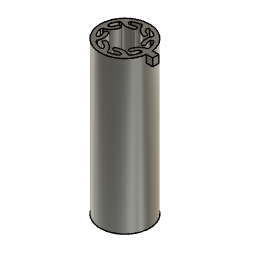
Linear_Bearing_V1.1 v1 (Autodesk Fusion 360 design; units mm, degrees)
Autodesk Fusion 360 part; units mm, degrees
sketch "Sketch1" plane through (0, 0, 0) normal (0, 0, 1) x (1, 0, 0)
  circle A0 centre (0, 0) radius 1.625
  spline S0 degree 5 poles (1.3709, -0.1056) (1.3505, -0.1114) (1.3112, -0.1235) (1.2571, -0.1431) (1.195, -0.1719) (1.1338, -0.2127) (1.088, -0.2577) (1.056, -0.3063) (1.0348, -0.3573) (1.0195, -0.4088) (1.0044, -0.4583) (0.984, -0.5029) (0.9544, -0.5399) (0.9148, -0.5662) (0.8686, -0.5794) (0.8219, -0.5775) (0.7819, -0.5594) (0.755, -0.5253) (0.7447, -0.4768) (0.751, -0.4174) (0.7717, -0.351) (0.8032, -0.2822) (0.8417, -0.2149) (0.8842, -0.1519) (0.9289, -0.0947) (0.9753, -0.0437) (1.0232, 0.0013) (1.0731, 0.0411) (1.1254, 0.0764) (1.1804, 0.1076) (1.2383, 0.135) (1.2869, 0.154) (1.3246, 0.1667) (1.3504, 0.1744) (1.3634, 0.1781) knots 0 0 0 0 0 0 0.033333 0.066667 0.1 0.133333 0.166667 0.2 0.233333 0.266667 0.3 0.333333 0.366667 0.4 0.433333 0.466667 0.5 0.533333 0.566667 0.6 0.633333 0.666667 0.7 0.733333 0.766667 0.8 0.833333 0.866667 0.9 0.933333 0.966667 1 1 1 1 1 1
  spline S1 degree 5 poles (1.0441, 0.8947) (1.0337, 0.8761) (1.0145, 0.8398) (0.9901, 0.7878) (0.9666, 0.7234) (0.9521, 0.6513) (0.9516, 0.5871) (0.9633, 0.5301) (0.9844, 0.479) (1.01, 0.4319) (1.0343, 0.3862) (1.0514, 0.3401) (1.0566, 0.2931) (1.0472, 0.2465) (1.0239, 0.2045) (0.9895, 0.1728) (0.9485, 0.1573) (0.9053, 0.1624) (0.8637, 0.1894) (0.8261, 0.2359) (0.7939, 0.2974) (0.7675, 0.3684) (0.7471, 0.4432) (0.7326, 0.5178) (0.7238, 0.5899) (0.7206, 0.6587) (0.7226, 0.7245) (0.7297, 0.7879) (0.7418, 0.8498) (0.7586, 0.9108) (0.7802, 0.971) (0.8011, 1.0188) (0.8188, 1.0545) (0.8315, 1.0782) (0.8381, 1.09) knots 0 0 0 0 0 0 0.033333 0.066667 0.1 0.133333 0.166667 0.2 0.233333 0.266667 0.3 0.333333 0.366667 0.4 0.433333 0.466667 0.5 0.533333 0.566667 0.6 0.633333 0.666667 0.7 0.733333 0.766667 0.8 0.833333 0.866667 0.9 0.933333 0.966667 1 1 1 1 1 1
  spline S2 degree 5 poles (0.1056, 1.3709) (0.1114, 1.3505) (0.1235, 1.3112) (0.1431, 1.2571) (0.1719, 1.195) (0.2127, 1.1338) (0.2577, 1.088) (0.3063, 1.056) (0.3573, 1.0348) (0.4088, 1.0195) (0.4583, 1.0044) (0.5029, 0.984) (0.5399, 0.9544) (0.5662, 0.9148) (0.5794, 0.8686) (0.5775, 0.8219) (0.5594, 0.7819) (0.5253, 0.755) (0.4768, 0.7447) (0.4174, 0.751) (0.351, 0.7717) (0.2822, 0.8032) (0.2149, 0.8417) (0.1519, 0.8842) (0.0947, 0.9289) (0.0437, 0.9753) (-0.0013, 1.0232) (-0.0411, 1.0731) (-0.0764, 1.1254) (-0.1076, 1.1804) (-0.135, 1.2383) (-0.154, 1.2869) (-0.1667, 1.3246) (-0.1744, 1.3504) (-0.1781, 1.3634) knots 0 0 0 0 0 0 0.033333 0.066667 0.1 0.133333 0.166667 0.2 0.233333 0.266667 0.3 0.333333 0.366667 0.4 0.433333 0.466667 0.5 0.533333 0.566667 0.6 0.633333 0.666667 0.7 0.733333 0.766667 0.8 0.833333 0.866667 0.9 0.933333 0.966667 1 1 1 1 1 1
  spline S3 degree 5 poles (-0.8947, 1.0441) (-0.8761, 1.0337) (-0.8398, 1.0145) (-0.7878, 0.9901) (-0.7234, 0.9666) (-0.6513, 0.9521) (-0.5871, 0.9516) (-0.5301, 0.9633) (-0.479, 0.9844) (-0.4319, 1.01) (-0.3862, 1.0343) (-0.3401, 1.0514) (-0.2931, 1.0566) (-0.2465, 1.0472) (-0.2045, 1.0239) (-0.1728, 0.9895) (-0.1573, 0.9485) (-0.1624, 0.9053) (-0.1894, 0.8637) (-0.2359, 0.8261) (-0.2974, 0.7939) (-0.3684, 0.7675) (-0.4432, 0.7471) (-0.5178, 0.7326) (-0.5899, 0.7238) (-0.6587, 0.7206) (-0.7245, 0.7226) (-0.7879, 0.7297) (-0.8498, 0.7418) (-0.9108, 0.7586) (-0.971, 0.7802) (-1.0188, 0.8011) (-1.0545, 0.8188) (-1.0782, 0.8315) (-1.09, 0.8381) knots 0 0 0 0 0 0 0.033333 0.066667 0.1 0.133333 0.166667 0.2 0.233333 0.266667 0.3 0.333333 0.366667 0.4 0.433333 0.466667 0.5 0.533333 0.566667 0.6 0.633333 0.666667 0.7 0.733333 0.766667 0.8 0.833333 0.866667 0.9 0.933333 0.966667 1 1 1 1 1 1
  spline S4 degree 5 poles (-1.3709, 0.1056) (-1.3505, 0.1114) (-1.3112, 0.1235) (-1.2571, 0.1431) (-1.195, 0.1719) (-1.1338, 0.2127) (-1.088, 0.2577) (-1.056, 0.3063) (-1.0348, 0.3573) (-1.0195, 0.4088) (-1.0044, 0.4583) (-0.984, 0.5029) (-0.9544, 0.5399) (-0.9148, 0.5662) (-0.8686, 0.5794) (-0.8219, 0.5775) (-0.7819, 0.5594) (-0.755, 0.5253) (-0.7447, 0.4768) (-0.751, 0.4174) (-0.7717, 0.351) (-0.8032, 0.2822) (-0.8417, 0.2149) (-0.8842, 0.1519) (-0.9289, 0.0947) (-0.9753, 0.0437) (-1.0232, -0.0013) (-1.0731, -0.0411) (-1.1254, -0.0764) (-1.1804, -0.1076) (-1.2383, -0.135) (-1.2869, -0.154) (-1.3246, -0.1667) (-1.3504, -0.1744) (-1.3634, -0.1781) knots 0 0 0 0 0 0 0.033333 0.066667 0.1 0.133333 0.166667 0.2 0.233333 0.266667 0.3 0.333333 0.366667 0.4 0.433333 0.466667 0.5 0.533333 0.566667 0.6 0.633333 0.666667 0.7 0.733333 0.766667 0.8 0.833333 0.866667 0.9 0.933333 0.966667 1 1 1 1 1 1
  spline S5 degree 5 poles (-1.0441, -0.8947) (-1.0337, -0.8761) (-1.0145, -0.8398) (-0.9901, -0.7878) (-0.9666, -0.7234) (-0.9521, -0.6513) (-0.9516, -0.5871) (-0.9633, -0.5301) (-0.9844, -0.479) (-1.01, -0.4319) (-1.0343, -0.3862) (-1.0514, -0.3401) (-1.0566, -0.2931) (-1.0472, -0.2465) (-1.0239, -0.2045) (-0.9895, -0.1728) (-0.9485, -0.1573) (-0.9053, -0.1624) (-0.8637, -0.1894) (-0.8261, -0.2359) (-0.7939, -0.2974) (-0.7675, -0.3684) (-0.7471, -0.4432) (-0.7326, -0.5178) (-0.7238, -0.5899) (-0.7206, -0.6587) (-0.7226, -0.7245) (-0.7297, -0.7879) (-0.7418, -0.8498) (-0.7586, -0.9108) (-0.7802, -0.971) (-0.8011, -1.0188) (-0.8188, -1.0545) (-0.8315, -1.0782) (-0.8381, -1.09) knots 0 0 0 0 0 0 0.033333 0.066667 0.1 0.133333 0.166667 0.2 0.233333 0.266667 0.3 0.333333 0.366667 0.4 0.433333 0.466667 0.5 0.533333 0.566667 0.6 0.633333 0.666667 0.7 0.733333 0.766667 0.8 0.833333 0.866667 0.9 0.933333 0.966667 1 1 1 1 1 1
  spline S6 degree 5 poles (-0.1056, -1.3709) (-0.1114, -1.3505) (-0.1235, -1.3112) (-0.1431, -1.2571) (-0.1719, -1.195) (-0.2127, -1.1338) (-0.2577, -1.088) (-0.3063, -1.056) (-0.3573, -1.0348) (-0.4088, -1.0195) (-0.4583, -1.0044) (-0.5029, -0.984) (-0.5399, -0.9544) (-0.5662, -0.9148) (-0.5794, -0.8686) (-0.5775, -0.8219) (-0.5594, -0.7819) (-0.5253, -0.755) (-0.4768, -0.7447) (-0.4174, -0.751) (-0.351, -0.7717) (-0.2822, -0.8032) (-0.2149, -0.8417) (-0.1519, -0.8842) (-0.0947, -0.9289) (-0.0437, -0.9753) (0.0013, -1.0232) (0.0411, -1.0731) (0.0764, -1.1254) (0.1076, -1.1804) (0.135, -1.2383) (0.154, -1.2869) (0.1667, -1.3246) (0.1744, -1.3504) (0.1781, -1.3634) knots 0 0 0 0 0 0 0.033333 0.066667 0.1 0.133333 0.166667 0.2 0.233333 0.266667 0.3 0.333333 0.366667 0.4 0.433333 0.466667 0.5 0.533333 0.566667 0.6 0.633333 0.666667 0.7 0.733333 0.766667 0.8 0.833333 0.866667 0.9 0.933333 0.966667 1 1 1 1 1 1
  spline S7 degree 5 poles (0.8947, -1.0441) (0.8761, -1.0337) (0.8398, -1.0145) (0.7878, -0.9901) (0.7234, -0.9666) (0.6513, -0.9521) (0.5871, -0.9516) (0.5301, -0.9633) (0.479, -0.9844) (0.4319, -1.01) (0.3862, -1.0343) (0.3401, -1.0514) (0.2931, -1.0566) (0.2465, -1.0472) (0.2045, -1.0239) (0.1728, -0.9895) (0.1573, -0.9485) (0.1624, -0.9053) (0.1894, -0.8637) (0.2359, -0.8261) (0.2974, -0.7939) (0.3684, -0.7675) (0.4432, -0.7471) (0.5178, -0.7326) (0.5899, -0.7238) (0.6587, -0.7206) (0.7245, -0.7226) (0.7879, -0.7297) (0.8498, -0.7418) (0.9108, -0.7586) (0.971, -0.7802) (1.0188, -0.8011) (1.0545, -0.8188) (1.0782, -0.8315) (1.09, -0.8381) knots 0 0 0 0 0 0 0.033333 0.066667 0.1 0.133333 0.166667 0.2 0.233333 0.266667 0.3 0.333333 0.366667 0.4 0.433333 0.466667 0.5 0.533333 0.566667 0.6 0.633333 0.666667 0.7 0.733333 0.766667 0.8 0.833333 0.866667 0.9 0.933333 0.966667 1 1 1 1 1 1
  arc A1 (1.3634, 0.1781) -> (1.0441, 0.8947) centre (0, 0) ccw
  arc A2 (0.8381, 1.09) -> (0.1056, 1.3709) centre (0, 0) ccw
  arc A3 (-0.1781, 1.3634) -> (-0.8947, 1.0441) centre (0, 0) ccw
  arc A4 (-1.09, 0.8381) -> (-1.3709, 0.1056) centre (0, 0) ccw
  arc A5 (-1.3634, -0.1781) -> (-1.0441, -0.8947) centre (0, 0) ccw
  arc A6 (-0.8381, -1.09) -> (-0.1056, -1.3709) centre (0, 0) ccw
  arc A7 (0.1781, -1.3634) -> (0.8947, -1.0441) centre (0, 0) ccw
  arc A8 (1.09, -0.8381) -> (1.3709, -0.1056) centre (0, 0) ccw
  point P0 (1.0505, -0.323)
  point P1 (0.9486, -0.5402)
  point P2 (0.7669, -0.5357)
  point P3 (0.8289, -0.2388)
  point P4 (1.0683, 0.0359)
  point P5 (0.9713, 0.5144)
  point P6 (1.0527, 0.2888)
  point P7 (0.9211, 0.1635)
  point P8 (0.755, 0.4173)
  point P9 (0.73, 0.7808)
  point P10 (0.323, 1.0505)
  point P11 (0.5402, 0.9486)
  point P12 (0.5357, 0.7669)
  point P13 (0.2388, 0.8289)
  point P14 (-0.0359, 1.0683)
  point P15 (-0.5144, 0.9713)
  point P16 (-0.2888, 1.0527)
  point P17 (-0.1635, 0.9211)
  point P18 (-0.4173, 0.755)
  point P19 (-0.7808, 0.73)
  point P20 (-1.0505, 0.323)
  point P21 (-0.9486, 0.5402)
  point P22 (-0.7669, 0.5357)
  point P23 (-0.8289, 0.2388)
  point P24 (-1.0683, -0.0359)
  point P25 (-0.9713, -0.5144)
  point P26 (-1.0527, -0.2888)
  point P27 (-0.9211, -0.1635)
  point P28 (-0.755, -0.4173)
  point P29 (-0.73, -0.7808)
  point P30 (-0.323, -1.0505)
  point P31 (-0.5402, -0.9486)
  point P32 (-0.5357, -0.7669)
  point P33 (-0.2388, -0.8289)
  point P34 (0.0359, -1.0683)
  point P35 (0.5144, -0.9713)
  point P36 (0.2888, -1.0527)
  point P37 (0.1635, -0.9211)
  point P38 (0.4173, -0.755)
  point P39 (0.7808, -0.73)
  dimension "d1" = 3.25
  dimension "d2" = 2.75
  dimension "d4" = 360
  constraint coincident A0.centre A1.centre
  constraint concentric A1 A2
  constraint concentric A2 A3
  constraint concentric A3 A4
  constraint concentric A4 A5
  constraint concentric A5 A6
  constraint concentric A6 A7
  constraint concentric A7 A8
  measures "d1" diameter of A0
  measures "d2" diameter of A1
extrude "Extrude1" add sketch "Sketch1" along normal blind 10
fillet "Fillet1" radius 0.1 16 edges at (-1.09, 0.8381, 5) (-0.8947, 1.0441, 5) (-1.3634, -0.1781, 5) (-1.3709, 0.1056, 5) (-0.1781, 1.3634, 5) (0.8381, 1.09, 5) (1.3709, -0.1056, 5) (0.1056, 1.3709, 5) (1.0441, 0.8947, 5) (1.3634, 0.1781, 5) (1.09, -0.8381, 5) (0.8947, -1.0441, 5) (0.1781, -1.3634, 5) (-1.0441, -0.8947, 5) (-0.8381, -1.09, 5) (-0.1056, -1.3709, 5)
sketch "Sketch2" plane through (0, 0, 10) normal (0, 0, 1) x (-1, 0, 0)
  arc A0 (-1.1419, 0.7659) -> (-1.346, 0.2807) centre (0, 0) ccw
  spline S0 degree 3 poles (-1.0172, 0.8011) (-1.029, 0.8065) (-1.0418, 0.8096) (-1.0678, 0.8107) (-1.0808, 0.8087) (-1.1029, 0.8006) (-1.1122, 0.7955) (-1.1288, 0.7825) (-1.136, 0.7747) (-1.1419, 0.7659) knots 0 0 0 0 0.003906 0.003906 0.007813 0.007813 0.010976 0.010976 0.01414 0.01414 0.01414 0.01414
  spline S1 degree 5 poles (-1.0172, 0.8011) (-1.0079, 0.7969) (-0.9867, 0.7875) (-0.9535, 0.7739) (-0.908, 0.7579) (-0.8498, 0.7418) (-0.7879, 0.7297) (-0.7245, 0.7226) (-0.6587, 0.7206) (-0.5899, 0.7238) (-0.5178, 0.7326) (-0.4432, 0.7471) (-0.3684, 0.7675) (-0.2974, 0.7939) (-0.2359, 0.8261) (-0.1894, 0.8637) (-0.1624, 0.9053) (-0.1573, 0.9485) (-0.1728, 0.9895) (-0.2045, 1.0239) (-0.2465, 1.0472) (-0.2931, 1.0566) (-0.3401, 1.0514) (-0.3862, 1.0343) (-0.4319, 1.01) (-0.479, 0.9844) (-0.5301, 0.9633) (-0.5871, 0.9516) (-0.6386, 0.952) (-0.6809, 0.9586) (-0.7108, 0.966) (-0.7262, 0.9705) (-0.7264, 0.9706) knots -0.959103 -0.959103 -0.959103 -0.959103 -0.959103 -0.959103 -0.933333 -0.9 -0.866667 -0.833333 -0.8 -0.766667 -0.733333 -0.7 -0.666667 -0.633333 -0.6 -0.566667 -0.533333 -0.5 -0.466667 -0.433333 -0.4 -0.366667 -0.333333 -0.3 -0.266667 -0.233333 -0.2 -0.166667 -0.133333 -0.1 -0.066667 -0.066274 -0.066274 -0.066274 -0.066274 -0.066274 -0.066274
  spline S2 degree 3 poles (-0.7533, 1.1503) (-0.7642, 1.1431) (-0.7736, 1.1339) (-0.7884, 1.1125) (-0.7936, 1.1004) (-0.799, 1.0749) (-0.7993, 1.0618) (-0.7947, 1.0362) (-0.7899, 1.0239) (-0.7764, 1.0027) (-0.7682, 0.9938) (-0.7489, 0.9794) (-0.738, 0.9739) (-0.7264, 0.9706) knots 0 0 0 0 0.003906 0.003906 0.007813 0.007813 0.011719 0.011719 0.015626 0.015626 0.019244 0.019244 0.022863 0.022863 0.022863 0.022863
  arc A1 (-0.2659, 1.3491) -> (-0.7533, 1.1503) centre (0, 0) ccw
  spline S3 degree 3 poles (-0.1528, 1.2857) (-0.1573, 1.2979) (-0.1642, 1.3091) (-0.1818, 1.3283) (-0.1924, 1.336) (-0.2138, 1.346) (-0.224, 1.3489) (-0.2449, 1.3515) (-0.2555, 1.3511) (-0.2659, 1.3491) knots 0 0 0 0 0.003906 0.003906 0.007813 0.007813 0.010976 0.010976 0.01414 0.01414 0.01414 0.01414
  spline S4 degree 5 poles (-0.1528, 1.2857) (-0.1492, 1.2762) (-0.1409, 1.2546) (-0.127, 1.2215) (-0.1061, 1.1779) (-0.0764, 1.1254) (-0.0411, 1.0731) (-0.0013, 1.0232) (0.0437, 0.9753) (0.0947, 0.9289) (0.1519, 0.8842) (0.2149, 0.8417) (0.2822, 0.8032) (0.351, 0.7717) (0.4174, 0.751) (0.4768, 0.7447) (0.5253, 0.755) (0.5594, 0.7819) (0.5775, 0.8219) (0.5794, 0.8686) (0.5662, 0.9148) (0.5399, 0.9544) (0.5029, 0.984) (0.4583, 1.0044) (0.4088, 1.0195) (0.3573, 1.0348) (0.3063, 1.056) (0.2577, 1.088) (0.2216, 1.1247) (0.1964, 1.1593) (0.1805, 1.1857) (0.1727, 1.1998) (0.1726, 1.1999) knots -0.959103 -0.959103 -0.959103 -0.959103 -0.959103 -0.959103 -0.933333 -0.9 -0.866667 -0.833333 -0.8 -0.766667 -0.733333 -0.7 -0.666667 -0.633333 -0.6 -0.566667 -0.533333 -0.5 -0.466667 -0.433333 -0.4 -0.366667 -0.333333 -0.3 -0.266667 -0.233333 -0.2 -0.166667 -0.133333 -0.1 -0.066667 -0.066274 -0.066274 -0.066274 -0.066274 -0.066274 -0.066274
  spline S5 degree 3 poles (0.2807, 1.346) (0.2679, 1.3487) (0.2548, 1.3488) (0.2292, 1.3441) (0.217, 1.3392) (0.1951, 1.3251) (0.1856, 1.316) (0.1707, 1.2946) (0.1655, 1.2826) (0.16, 1.2581) (0.1596, 1.2459) (0.163, 1.222) (0.1668, 1.2105) (0.1726, 1.1999) knots 0 0 0 0 0.003906 0.003906 0.007813 0.007813 0.011719 0.011719 0.015626 0.015626 0.019244 0.019244 0.022863 0.022863 0.022863 0.022863
  arc A2 (0.7659, 1.1419) -> (0.2807, 1.346) centre (0, 0) ccw
  spline S6 degree 3 poles (0.8011, 1.0172) (0.8065, 1.029) (0.8096, 1.0418) (0.8107, 1.0678) (0.8087, 1.0808) (0.8006, 1.1029) (0.7955, 1.1122) (0.7825, 1.1288) (0.7747, 1.136) (0.7659, 1.1419) knots 0 0 0 0 0.003906 0.003906 0.007813 0.007813 0.010976 0.010976 0.01414 0.01414 0.01414 0.01414
  spline S7 degree 5 poles (0.8011, 1.0172) (0.7969, 1.0079) (0.7875, 0.9867) (0.7739, 0.9535) (0.7579, 0.908) (0.7418, 0.8498) (0.7297, 0.7879) (0.7226, 0.7245) (0.7206, 0.6587) (0.7238, 0.5899) (0.7326, 0.5178) (0.7471, 0.4432) (0.7675, 0.3684) (0.7939, 0.2974) (0.8261, 0.2359) (0.8637, 0.1894) (0.9053, 0.1624) (0.9485, 0.1573) (0.9895, 0.1728) (1.0239, 0.2045) (1.0472, 0.2465) (1.0566, 0.2931) (1.0514, 0.3401) (1.0343, 0.3862) (1.01, 0.4319) (0.9844, 0.479) (0.9633, 0.5301) (0.9516, 0.5871) (0.952, 0.6386) (0.9586, 0.6809) (0.966, 0.7108) (0.9705, 0.7262) (0.9706, 0.7264) knots -0.959103 -0.959103 -0.959103 -0.959103 -0.959103 -0.959103 -0.933333 -0.9 -0.866667 -0.833333 -0.8 -0.766667 -0.733333 -0.7 -0.666667 -0.633333 -0.6 -0.566667 -0.533333 -0.5 -0.466667 -0.433333 -0.4 -0.366667 -0.333333 -0.3 -0.266667 -0.233333 -0.2 -0.166667 -0.133333 -0.1 -0.066667 -0.066274 -0.066274 -0.066274 -0.066274 -0.066274 -0.066274
  spline S8 degree 3 poles (1.1503, 0.7533) (1.1431, 0.7642) (1.1339, 0.7736) (1.1125, 0.7884) (1.1004, 0.7936) (1.0749, 0.799) (1.0618, 0.7993) (1.0362, 0.7947) (1.0239, 0.7899) (1.0027, 0.7764) (0.9938, 0.7682) (0.9794, 0.7489) (0.9739, 0.738) (0.9706, 0.7264) knots 0 0 0 0 0.003906 0.003906 0.007813 0.007813 0.011719 0.011719 0.015626 0.015626 0.019244 0.019244 0.022863 0.022863 0.022863 0.022863
  arc A3 (1.3491, 0.2659) -> (1.1503, 0.7533) centre (0, 0) ccw
  spline S9 degree 3 poles (1.2857, 0.1528) (1.2979, 0.1573) (1.3091, 0.1642) (1.3283, 0.1818) (1.336, 0.1924) (1.346, 0.2138) (1.3489, 0.224) (1.3515, 0.2449) (1.3511, 0.2555) (1.3491, 0.2659) knots 0 0 0 0 0.003906 0.003906 0.007813 0.007813 0.010976 0.010976 0.01414 0.01414 0.01414 0.01414
  spline S10 degree 5 poles (1.2857, 0.1528) (1.2762, 0.1492) (1.2546, 0.1409) (1.2215, 0.127) (1.1779, 0.1061) (1.1254, 0.0764) (1.0731, 0.0411) (1.0232, 0.0013) (0.9753, -0.0437) (0.9289, -0.0947) (0.8842, -0.1519) (0.8417, -0.2149) (0.8032, -0.2822) (0.7717, -0.351) (0.751, -0.4174) (0.7447, -0.4768) (0.755, -0.5253) (0.7819, -0.5594) (0.8219, -0.5775) (0.8686, -0.5794) (0.9148, -0.5662) (0.9544, -0.5399) (0.984, -0.5029) (1.0044, -0.4583) (1.0195, -0.4088) (1.0348, -0.3573) (1.056, -0.3063) (1.088, -0.2577) (1.1247, -0.2216) (1.1593, -0.1964) (1.1857, -0.1805) (1.1998, -0.1727) (1.1999, -0.1726) knots -0.959103 -0.959103 -0.959103 -0.959103 -0.959103 -0.959103 -0.933333 -0.9 -0.866667 -0.833333 -0.8 -0.766667 -0.733333 -0.7 -0.666667 -0.633333 -0.6 -0.566667 -0.533333 -0.5 -0.466667 -0.433333 -0.4 -0.366667 -0.333333 -0.3 -0.266667 -0.233333 -0.2 -0.166667 -0.133333 -0.1 -0.066667 -0.066274 -0.066274 -0.066274 -0.066274 -0.066274 -0.066274
  spline S11 degree 3 poles (1.346, -0.2807) (1.3487, -0.2679) (1.3488, -0.2548) (1.3441, -0.2292) (1.3392, -0.217) (1.3251, -0.1951) (1.316, -0.1856) (1.2946, -0.1707) (1.2826, -0.1655) (1.2581, -0.16) (1.2459, -0.1596) (1.222, -0.163) (1.2105, -0.1668) (1.1999, -0.1726) knots 0 0 0 0 0.003906 0.003906 0.007813 0.007813 0.011719 0.011719 0.015626 0.015626 0.019244 0.019244 0.022863 0.022863 0.022863 0.022863
  arc A4 (1.1419, -0.7659) -> (1.346, -0.2807) centre (0, 0) ccw
  spline S12 degree 3 poles (1.0172, -0.8011) (1.029, -0.8065) (1.0418, -0.8096) (1.0678, -0.8107) (1.0808, -0.8087) (1.1029, -0.8006) (1.1122, -0.7955) (1.1288, -0.7825) (1.136, -0.7747) (1.1419, -0.7659) knots 0 0 0 0 0.003906 0.003906 0.007813 0.007813 0.010976 0.010976 0.01414 0.01414 0.01414 0.01414
  spline S13 degree 5 poles (1.0172, -0.8011) (1.0079, -0.7969) (0.9867, -0.7875) (0.9535, -0.7739) (0.908, -0.7579) (0.8498, -0.7418) (0.7879, -0.7297) (0.7245, -0.7226) (0.6587, -0.7206) (0.5899, -0.7238) (0.5178, -0.7326) (0.4432, -0.7471) (0.3684, -0.7675) (0.2974, -0.7939) (0.2359, -0.8261) (0.1894, -0.8637) (0.1624, -0.9053) (0.1573, -0.9485) (0.1728, -0.9895) (0.2045, -1.0239) (0.2465, -1.0472) (0.2931, -1.0566) (0.3401, -1.0514) (0.3862, -1.0343) (0.4319, -1.01) (0.479, -0.9844) (0.5301, -0.9633) (0.5871, -0.9516) (0.6386, -0.952) (0.6809, -0.9586) (0.7108, -0.966) (0.7262, -0.9705) (0.7264, -0.9706) knots -0.959103 -0.959103 -0.959103 -0.959103 -0.959103 -0.959103 -0.933333 -0.9 -0.866667 -0.833333 -0.8 -0.766667 -0.733333 -0.7 -0.666667 -0.633333 -0.6 -0.566667 -0.533333 -0.5 -0.466667 -0.433333 -0.4 -0.366667 -0.333333 -0.3 -0.266667 -0.233333 -0.2 -0.166667 -0.133333 -0.1 -0.066667 -0.066274 -0.066274 -0.066274 -0.066274 -0.066274 -0.066274
  spline S14 degree 3 poles (0.7533, -1.1503) (0.7642, -1.1431) (0.7736, -1.1339) (0.7884, -1.1125) (0.7936, -1.1004) (0.799, -1.0749) (0.7993, -1.0618) (0.7947, -1.0362) (0.7899, -1.0239) (0.7764, -1.0027) (0.7682, -0.9938) (0.7489, -0.9794) (0.738, -0.9739) (0.7264, -0.9706) knots 0 0 0 0 0.003906 0.003906 0.007813 0.007813 0.011719 0.011719 0.015626 0.015626 0.019244 0.019244 0.022863 0.022863 0.022863 0.022863
  arc A5 (0.2659, -1.3491) -> (0.7533, -1.1503) centre (0, 0) ccw
  spline S15 degree 3 poles (0.1528, -1.2857) (0.1573, -1.2979) (0.1642, -1.3091) (0.1818, -1.3283) (0.1924, -1.336) (0.2138, -1.346) (0.224, -1.3489) (0.2449, -1.3515) (0.2555, -1.3511) (0.2659, -1.3491) knots 0 0 0 0 0.003906 0.003906 0.007813 0.007813 0.010976 0.010976 0.01414 0.01414 0.01414 0.01414
  spline S16 degree 5 poles (0.1528, -1.2857) (0.1492, -1.2762) (0.1409, -1.2546) (0.127, -1.2215) (0.1061, -1.1779) (0.0764, -1.1254) (0.0411, -1.0731) (0.0013, -1.0232) (-0.0437, -0.9753) (-0.0947, -0.9289) (-0.1519, -0.8842) (-0.2149, -0.8417) (-0.2822, -0.8032) (-0.351, -0.7717) (-0.4174, -0.751) (-0.4768, -0.7447) (-0.5253, -0.755) (-0.5594, -0.7819) (-0.5775, -0.8219) (-0.5794, -0.8686) (-0.5662, -0.9148) (-0.5399, -0.9544) (-0.5029, -0.984) (-0.4583, -1.0044) (-0.4088, -1.0195) (-0.3573, -1.0348) (-0.3063, -1.056) (-0.2577, -1.088) (-0.2216, -1.1247) (-0.1964, -1.1593) (-0.1805, -1.1857) (-0.1727, -1.1998) (-0.1726, -1.1999) knots -0.959103 -0.959103 -0.959103 -0.959103 -0.959103 -0.959103 -0.933333 -0.9 -0.866667 -0.833333 -0.8 -0.766667 -0.733333 -0.7 -0.666667 -0.633333 -0.6 -0.566667 -0.533333 -0.5 -0.466667 -0.433333 -0.4 -0.366667 -0.333333 -0.3 -0.266667 -0.233333 -0.2 -0.166667 -0.133333 -0.1 -0.066667 -0.066274 -0.066274 -0.066274 -0.066274 -0.066274 -0.066274
  spline S17 degree 3 poles (-0.2807, -1.346) (-0.2679, -1.3487) (-0.2548, -1.3488) (-0.2292, -1.3441) (-0.217, -1.3392) (-0.1951, -1.3251) (-0.1856, -1.316) (-0.1707, -1.2946) (-0.1655, -1.2826) (-0.16, -1.2581) (-0.1596, -1.2459) (-0.163, -1.222) (-0.1668, -1.2105) (-0.1726, -1.1999) knots 0 0 0 0 0.003906 0.003906 0.007813 0.007813 0.011719 0.011719 0.015626 0.015626 0.019244 0.019244 0.022863 0.022863 0.022863 0.022863
  arc A6 (-0.7659, -1.1419) -> (-0.2807, -1.346) centre (0, 0) ccw
  spline S18 degree 3 poles (-0.8011, -1.0172) (-0.8065, -1.029) (-0.8096, -1.0418) (-0.8107, -1.0678) (-0.8087, -1.0808) (-0.8006, -1.1029) (-0.7955, -1.1122) (-0.7825, -1.1288) (-0.7747, -1.136) (-0.7659, -1.1419) knots 0 0 0 0 0.003906 0.003906 0.007813 0.007813 0.010976 0.010976 0.01414 0.01414 0.01414 0.01414
  spline S19 degree 5 poles (-0.8011, -1.0172) (-0.7969, -1.0079) (-0.7875, -0.9867) (-0.7739, -0.9535) (-0.7579, -0.908) (-0.7418, -0.8498) (-0.7297, -0.7879) (-0.7226, -0.7245) (-0.7206, -0.6587) (-0.7238, -0.5899) (-0.7326, -0.5178) (-0.7471, -0.4432) (-0.7675, -0.3684) (-0.7939, -0.2974) (-0.8261, -0.2359) (-0.8637, -0.1894) (-0.9053, -0.1624) (-0.9485, -0.1573) (-0.9895, -0.1728) (-1.0239, -0.2045) (-1.0472, -0.2465) (-1.0566, -0.2931) (-1.0514, -0.3401) (-1.0343, -0.3862) (-1.01, -0.4319) (-0.9844, -0.479) (-0.9633, -0.5301) (-0.9516, -0.5871) (-0.952, -0.6386) (-0.9586, -0.6809) (-0.966, -0.7108) (-0.9705, -0.7262) (-0.9706, -0.7264) knots -0.959103 -0.959103 -0.959103 -0.959103 -0.959103 -0.959103 -0.933333 -0.9 -0.866667 -0.833333 -0.8 -0.766667 -0.733333 -0.7 -0.666667 -0.633333 -0.6 -0.566667 -0.533333 -0.5 -0.466667 -0.433333 -0.4 -0.366667 -0.333333 -0.3 -0.266667 -0.233333 -0.2 -0.166667 -0.133333 -0.1 -0.066667 -0.066274 -0.066274 -0.066274 -0.066274 -0.066274 -0.066274
  spline S20 degree 3 poles (-1.1503, -0.7533) (-1.1431, -0.7642) (-1.1339, -0.7736) (-1.1125, -0.7884) (-1.1004, -0.7936) (-1.0749, -0.799) (-1.0618, -0.7993) (-1.0362, -0.7947) (-1.0239, -0.7899) (-1.0027, -0.7764) (-0.9938, -0.7682) (-0.9794, -0.7489) (-0.9739, -0.738) (-0.9706, -0.7264) knots 0 0 0 0 0.003906 0.003906 0.007813 0.007813 0.011719 0.011719 0.015626 0.015626 0.019244 0.019244 0.022863 0.022863 0.022863 0.022863
  arc A7 (-1.3491, -0.2659) -> (-1.1503, -0.7533) centre (0, 0) ccw
  spline S21 degree 3 poles (-1.2857, -0.1528) (-1.2979, -0.1573) (-1.3091, -0.1642) (-1.3283, -0.1818) (-1.336, -0.1924) (-1.346, -0.2138) (-1.3489, -0.224) (-1.3515, -0.2449) (-1.3511, -0.2555) (-1.3491, -0.2659) knots 0 0 0 0 0.003906 0.003906 0.007813 0.007813 0.010976 0.010976 0.01414 0.01414 0.01414 0.01414
  spline S22 degree 5 poles (-1.2857, -0.1528) (-1.2762, -0.1492) (-1.2546, -0.1409) (-1.2215, -0.127) (-1.1779, -0.1061) (-1.1254, -0.0764) (-1.0731, -0.0411) (-1.0232, -0.0013) (-0.9753, 0.0437) (-0.9289, 0.0947) (-0.8842, 0.1519) (-0.8417, 0.2149) (-0.8032, 0.2822) (-0.7717, 0.351) (-0.751, 0.4174) (-0.7447, 0.4768) (-0.755, 0.5253) (-0.7819, 0.5594) (-0.8219, 0.5775) (-0.8686, 0.5794) (-0.9148, 0.5662) (-0.9544, 0.5399) (-0.984, 0.5029) (-1.0044, 0.4583) (-1.0195, 0.4088) (-1.0348, 0.3573) (-1.056, 0.3063) (-1.088, 0.2577) (-1.1247, 0.2216) (-1.1593, 0.1964) (-1.1857, 0.1805) (-1.1998, 0.1727) (-1.1999, 0.1726) knots -0.959103 -0.959103 -0.959103 -0.959103 -0.959103 -0.959103 -0.933333 -0.9 -0.866667 -0.833333 -0.8 -0.766667 -0.733333 -0.7 -0.666667 -0.633333 -0.6 -0.566667 -0.533333 -0.5 -0.466667 -0.433333 -0.4 -0.366667 -0.333333 -0.3 -0.266667 -0.233333 -0.2 -0.166667 -0.133333 -0.1 -0.066667 -0.066274 -0.066274 -0.066274 -0.066274 -0.066274 -0.066274
  spline S23 degree 3 poles (-1.346, 0.2807) (-1.3487, 0.2679) (-1.3488, 0.2548) (-1.3441, 0.2292) (-1.3392, 0.217) (-1.3251, 0.1951) (-1.316, 0.1856) (-1.2946, 0.1707) (-1.2826, 0.1655) (-1.2581, 0.16) (-1.2459, 0.1596) (-1.222, 0.163) (-1.2105, 0.1668) (-1.1999, 0.1726) knots 0 0 0 0 0.003906 0.003906 0.007813 0.007813 0.011719 0.011719 0.015626 0.015626 0.019244 0.019244 0.022863 0.022863 0.022863 0.022863
  circle A8 centre (0, 0) radius 1.625
  line L0 (0, 0) -> (-1.625, 0)
  line L1 (-1.625, 0) -> (-1.8281, 0)
  line L2 (-1.625, 0.2031) -> (-2.0313, 0.2031)
  line L3 (-2.0313, 0.2031) -> (-2.0313, -0.2031)
  line L4 (-2.0313, -0.2031) -> (-1.625, -0.2031)
  line L5 (-1.625, -0.2031) -> (-1.625, 0.2031)
  line L6 (-1.625, 0.2031) -> (-2.0313, -0.2031) construction
  line L7 (-2.0313, 0.2031) -> (-1.625, -0.2031) construction
  line L8 (-1.625, 0.2031) -> (-1.6123, 0.2031)
  line L9 (-1.625, -0.2031) -> (-1.6123, -0.2031)
  point P0 (-1.8281, 0)
  dimension "d9" = 0.4063
  dimension "d10" = 0.4062
  constraint coincident A0.centre A1.centre
  constraint coincident A8 L0.end
  constraint horizontal L0
  constraint parallel L0 L1
  constraint horizontal L2
  constraint perpendicular L2 L3
  constraint parallel L2 L4
  constraint parallel L3 L5
  constraint coincident L6 P0
  constraint coincident L7 P0
  constraint coincident P0 L1.end
  constraint tangent A8 L5
  constraint coincident A8 L8.end
  constraint perpendicular L5 L8
  constraint coincident A8 L9.end
  constraint perpendicular L5 L9
  measures "d9" distance of L3.end L4.end
  measures "d10" distance of L2.end L3.end
extrude "Extrude2" add sketch "Sketch2" against normal blind 0.5 contours A8 L2 L3 L4 L5
scale "Scale1" factor 4.923077 about (1.6123, 0.2031, 10) bodies 1
